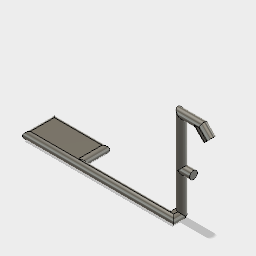
pegboard-hook-003a (Autodesk Fusion 360 design; units mm, degrees)
Autodesk Fusion 360 part; units mm, degrees
sketch "スケッチ3" plane through (0, 0, 0) normal (0, 1, 0) x (1, 0, 0)
  line L0 (5, -5) -> (10, -5)
  line L1 (10, -5) -> (10, -10)
  line L2 (10, -10) -> (5, -10)
  line L3 (5, -10) -> (5, -5)
  line L4 (-10, 0) -> (-5, 0)
  line L5 (-5, 0) -> (-5, 60)
  line L6 (-5, 60) -> (-10, 60)
  line L7 (-10, 60) -> (-10, 0)
  line L8 (10, 10) -> (10, 5)
  line L9 (10, 5) -> (17, 5)
  line L10 (17, 10) -> (10, 10)
  line L11 (-5, 55) -> (-10, 55)
  line L12 (-10, 55) -> (-10, 0)
  line L13 (-10, 0) -> (-5, 0)
  line L14 (-5, 0) -> (-5, 55)
  line L15 (17, 5) -> (17, 10)
  line L16 (22, 60) -> (5, 60)
  line L17 (5, 60) -> (5, 0)
  line L18 (5, 0) -> (10, 0)
  line L19 (10, 0) -> (10, 25)
  line L20 (10, 25) -> (15, 25)
  line L21 (15, 25) -> (15, 30)
  line L22 (15, 30) -> (10, 30)
  line L23 (10, 30) -> (10, 55)
  line L24 (10, 55) -> (17, 55)
  line L25 (17, 55) -> (22.6569, 49.3431)
  line L26 (22.6569, 49.3431) -> (27.6569, 54.3431)
  line L27 (27.6569, 54.3431) -> (22, 60)
  line L28 (5, 0) -> (15, 0)
  line L29 (15, 0) -> (15, 5)
  line L30 (15, 5) -> (10, 5)
  line L31 (10, 5) -> (10, 60)
  line L32 (10, 60) -> (5, 60)
  line L33 (5, 60) -> (5, 0)
  line L34 (-5, 5) -> (-5, 0)
  line L35 (-5, 0) -> (85, 0)
  line L36 (85, 0) -> (85, 5)
  line L37 (85, 5) -> (-5, 5)
  dimension "d4" = 5
  dimension "d5" = 5
  measures "d4" distance of L0 L2
  measures "d5" distance of L1 L3
  measures "d17" distance of L11.end
extrude "押し出し2" add sketch "スケッチ3" along normal blind 60 contours L0 L1 L2 L3
sketch "スケッチ4" plane through (10, 0, 0) normal (1, 0, 0) x (0, 0, -1)
  line L0 (-10, 0) -> (-5, 0)
  line L1 (-5, 0) -> (-5, 60)
  line L2 (-5, 60) -> (-10, 60)
  line L3 (-10, 60) -> (-10, 0)
  line L4 (-10, 60) -> (-5, 60)
  line L5 (-5, 60) -> (-5, 55)
  line L6 (-5, 55) -> (-10, 55)
  line L7 (-10, 55) -> (-10, 60)
  dimension "d10" = 5
  measures "d10" distance of L4 L6
extrude "押し出し4" add sketch "スケッチ4" along normal blind 12 contours L1 L2 L3 L4 L5 L6 L7
chamfer "面取り1" distance 5 angle 45 1 edges at (22, 55, 7.5)
extrude "押し出し9" add 2 faces at (22, 59.9997, 8.3333) (20.3337, 58.3327, 6.6667) along direction (0.707107, -0.707107, 0) blind 8
sketch "スケッチ5" plane through (0, 55, 0) normal (0, -1, 0) x (1, 0, 0)
  line L0 (10, 10) -> (10, 5)
  line L1 (10, 5) -> (17, 5)
  line L2 (17, 10) -> (10, 10)
  line L3 (17, 10) -> (12, 10)
  line L4 (12, 10) -> (12, 5)
  line L5 (12, 5) -> (17, 5)
  line L6 (17, 5) -> (17, 10)
  line L7 (17, 5) -> (17, 10)
  dimension "d13" = 5
  measures "d13" distance of L4 L6
sketch "スケッチ7" plane through (10, 0, 0) normal (1, 0, 0) x (0, 0, -1)
  line L0 (-5, 55) -> (-10, 55)
  line L1 (-10, 55) -> (-10, 0)
  line L2 (-10, 0) -> (-5, 0)
  line L3 (-5, 0) -> (-5, 55)
  line L4 (-10, 30) -> (-5, 30)
  line L5 (-5, 30) -> (-5, 25)
  line L6 (-5, 25) -> (-10, 25)
  line L7 (-10, 25) -> (-10, 30)
  dimension "d17" = 25
  dimension "d18" = 5
  measures "d17" distance of L0.end L4
  measures "d18" distance of L4 L6
extrude "押し出し6" add sketch "スケッチ7" along normal blind 5 contours L1 L3 L4 L5 L6 L7
sketch "スケッチ11" plane through (0, 0, 10) normal (0, 0, 1) x (1, 0, 0)
  line L0 (22, 60) -> (5, 60)
  line L1 (5, 60) -> (5, 0)
  line L2 (5, 0) -> (10, 0)
  line L3 (10, 0) -> (10, 25)
  line L4 (10, 25) -> (15, 25)
  line L5 (15, 25) -> (15, 30)
  line L6 (15, 30) -> (10, 30)
  line L7 (10, 30) -> (10, 55)
  line L8 (10, 55) -> (17, 55)
  line L9 (17, 55) -> (22.6569, 49.3431)
  line L10 (22.6569, 49.3431) -> (27.6569, 54.3431)
  line L11 (27.6569, 54.3431) -> (22, 60)
  line L12 (5, 0) -> (10, 0)
  line L13 (10, 0) -> (10, 5)
  line L14 (10, 5) -> (5, 5)
  line L15 (5, 5) -> (5, 0)
  dimension "d41" = 5
  measures "d41" distance of L12 L14
extrude "押し出し11" add sketch "スケッチ11" along normal blind 5 contours L1 L2 L3 L12 L13 L14 L15
sketch "スケッチ12" plane through (5, 0, 0) normal (-1, 0, 0) x (0, 0, 1)
  line L0 (5, 0) -> (15, 0)
  line L1 (15, 0) -> (15, 5)
  line L2 (15, 5) -> (10, 5)
  line L3 (10, 5) -> (10, 60)
  line L4 (10, 60) -> (5, 60)
  line L5 (5, 60) -> (5, 0)
  line L6 (15, 5) -> (10, 5)
  line L7 (10, 5) -> (10, 0)
  line L8 (10, 0) -> (15, 0)
  line L9 (15, 0) -> (15, 5)
  dimension "d44" = 5
  measures "d44" distance of L7 L9
extrude "押し出し12" add sketch "スケッチ12" along normal blind 90 contours L0 L1 L2 L6 L7 L8 L9
sketch "スケッチ13" plane through (0, 0, 10) normal (0, 0, -1) x (-1, 0, 0)
  line L0 (-5, 5) -> (-5, 0)
  line L1 (-5, 0) -> (85, 0)
  line L2 (85, 0) -> (85, 5)
  line L3 (85, 5) -> (-5, 5)
  line L4 (85, 5) -> (50, 5)
  line L5 (50, 5) -> (50, 0)
  line L6 (50, 0) -> (85, 0)
  line L7 (85, 0) -> (85, 5)
  dimension "d47" = 35
  measures "d47" distance of L5 L7
extrude "押し出し13" add sketch "スケッチ13" along normal blind 15 contours L1 L2 L3 L4 L5 L6 L7
fillet "フィレット9" radius 2.5 32 edges at (-37.5, 5, 15) (19.8284, 52.1716, 5) (24.8284, 57.1716, 5) (24.8284, 57.1716, 10) (19.8284, 52.1716, 10) (13.5, 60, 5) (13.5, 60, 10) (13.5, 55, 10) (10, 42.5, 10) (5, 32.5, 10) (5, 30, 5) (13.5, 55, 5) (10, 42.5, 5) (12.5, 30, 5) (12.5, 25, 5) (12.5, 25, 10) (12.5, 30, 10) (10, 15, 10) (10, 12.5, 5) (10, 5, 12.5) (10, 0, 10) (-37.5, 0, 15) (-22.5, 5, 10) (-22.5, 0, 10) (7.5, 0, 5) (5, 0, 7.5) (-50, 0, 2.5) (-67.5, 5, -5) (-67.5, 0, -5) (-85, 5, 5) (-85, 0, 5) (-50, 5, 2.5)
